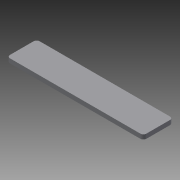
# Autodesk Inventor part: BumperWoodShort
Saved by Autodesk Inventor 2013 (Build 170138000, 138)
## iProperties
Created: 2014-02-13
Part Number: BumperWoodShort
Material: Generic
Document SubType Name: Modeling
Designer: 215152
Density: 1 g/cm^3
Author: 215152
Autodesk Inventor part; units mm, degrees
ref_plane "YZ Plane" through (0, 0, 0) normal (1, 0, 0) x (0, 1, 0)
ref_plane "XZ Plane" through (0, 0, 0) normal (0, 1, 0) x (-1, 0, 0)
ref_plane "XY Plane" through (0, 0, 0) normal (0, 0, 1) x (1, 0, 0)
sketch "Sketch1" plane through (0, 0, 0) normal (0, 1, 0) x (-1, 0, 0)
  line L0 (279.4, 63.5) -> (-279.4, 63.5)
  line L1 (-292.1, 50.8) -> (-292.1, -50.8)
  line L2 (-279.4, -63.5) -> (279.4, -63.5)
  line L3 (292.1, -50.8) -> (292.1, 50.8)
  line L4 (292.1, 63.5) -> (-292.1, -63.5) construction
  line L5 (-292.1, 63.5) -> (292.1, -63.5) construction
  arc A0 (279.4, -63.5) -> (292.1, -50.8) centre (279.4, -50.8) ccw
  arc A1 (292.1, 50.8) -> (279.4, 63.5) centre (279.4, 50.8) ccw
  arc A2 (-279.4, 63.5) -> (-292.1, 50.8) centre (-279.4, 50.8) ccw
  arc A3 (-292.1, -50.8) -> (-279.4, -63.5) centre (-279.4, -50.8) ccw
  point P0 (0, 0)
  dimension "d0" = 584.2
  dimension "d1" = 127
  dimension "d2" = 12.7
  constraints: 12 end point, 8 point on circle, 8 point on line, 8 tangent, 4 centre point, 3 equal radius, 2 midpoint, 2 parallel, 1 horizontal, 1 perpendicular
  measures "d0" distance of L5.end L4.end
  measures "d1" distance of L4.end L5.start
  measures "d2" radius of A0
extrude "Extrusion1" add sketch "Sketch1" along normal blind 19.05
body "Solid1"
